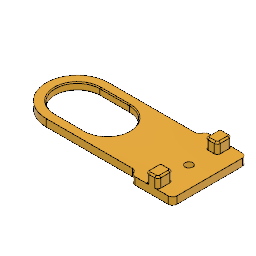
filament guide v6 (Autodesk Fusion 360 design; units mm, degrees)
Autodesk Fusion 360 part; units mm, degrees
sketch "Sketch1" plane through (0, 0, 0) normal (0, 1, 0) x (1, 0, 0)
  line L0 (0, 0) -> (-75, 0) construction
  circle A0 centre (-75, 0) radius 15
  circle A1 centre (-75, 0) radius 21
  circle A2 centre (-55, 0) radius 15
  line L1 (14, -25) -> (-14, -25)
  line L2 (-14, -25) -> (-14, 25)
  line L3 (-14, 25) -> (14, 25)
  line L4 (14, 25) -> (14, -25)
  line L5 (14, -25) -> (-14, 25) construction
  line L6 (-14, -25) -> (14, 25) construction
  line L7 (-14, 21) -> (-75, 21)
  line L8 (-14, -21) -> (-75, -21)
  line L9 (-75, 15) -> (-55, 15)
  line L10 (-75, -15) -> (-55, -15)
  circle A3 centre (0, 0) radius 2.6
  line L11 (15, -29.9919) -> (-15, -29.9919) construction
  line L12 (-15, -29.9919) -> (-15, 29.9919) construction
  line L13 (-15, 29.9919) -> (15, 29.9919) construction
  line L14 (15, 29.9919) -> (15, -29.9919) construction
  line L15 (15, -29.9919) -> (-15, 29.9919) construction
  line L16 (-15, -29.9919) -> (15, 29.9919) construction
  line L17 (-4.05, -25) -> (4.05, -25)
  line L18 (4.05, -25) -> (4.05, -15)
  line L19 (4.05, -15) -> (-4.05, -15)
  line L20 (-4.05, -15) -> (-4.05, -25)
  line L21 (0, -25) -> (0, 25) construction
  line L22 (4.05, 25) -> (4.05, 15)
  line L23 (4.05, 15) -> (-4.05, 15)
  line L24 (-4.05, 25) -> (4.05, 25)
  line L25 (-4.05, 15) -> (-4.05, 25)
  point P0 (-90, 0)
  point P1 (-40, 0)
  dimension "d1" = 30
  dimension "d3" = 30
  dimension "d4" = 42
  dimension "d5" = 50
  dimension "d6" = 28
  dimension "d9" = 5.2
  dimension "d20" = 30
  dimension "d23" = 75
  dimension "d24" = 25
  dimension "d25" = 10
  dimension "d26" = 8.1
  constraint horizontal L0
  constraint coincident A3.centre L0
  constraint coincident L0 A0.centre
  constraint coincident L0 A2.centre
  constraint perpendicular L1 L2
  constraint parallel L1 L3
  constraint parallel L2 L4
  constraint horizontal L1
  constraint coincident L5 L0.start
  constraint coincident L6 L0.start
  constraint coincident L0.start A3.centre
  constraint coincident L2 L7.start
  constraint coincident A1 L7.end
  constraint tangent A1 L7
  constraint horizontal L7
  constraint coincident L2 L8.start
  constraint coincident A1 L8.end
  constraint tangent A1 L8
  constraint horizontal L8
  constraint coincident A0 L9.start
  constraint coincident A2 L9.end
  constraint tangent A2 L9
  constraint horizontal L9
  constraint coincident A0 L10.start
  constraint coincident A2 L10.end
  constraint tangent A2 L10
  constraint horizontal L10
  constraint coincident A0 P0
  constraint coincident A2 P1
  constraint coincident L0 P0
  constraint coincident L0 P1
  constraint coincident L0.end A0.centre
  constraint perpendicular L11 L12
  constraint parallel L11 L13
  constraint parallel L12 L14
  constraint horizontal L11
  constraint coincident L15 L0.start
  constraint coincident L16 L0.start
  constraint concentric A0 A1
  constraint horizontal L17
  constraint vertical L18
  constraint horizontal L19
  constraint vertical L20
  constraint midpoint L1 L21.start
  constraint midpoint L3 L21.end
  constraint midpoint L17 L21.start
  constraint symmetric L0 L17.start L24.start
  constraint symmetric L0 L17.end L22.start
  constraint symmetric L0 L18.end L22.end
  constraint symmetric L0 L19.end L23.end
  measures "d1" diameter of A2
  measures "d3" diameter of A0
  measures "d4" diameter of A1
  measures "d5" distance of L1.end L2.end
  measures "d6" distance of L2.end L3.end
  measures "d9" diameter of A3
  measures "d20" distance of L11.start L11.end
  measures "d23" distance of P0 L12
  measures "d24" distance of P1 L12
  measures "d25" distance of L17.end L18.end
  measures "d26" distance of L17.start L17.end
extrude "Extrude1" add sketch "Sketch1" along normal blind 5 contours A0 A1 L9 L10 | A1 A2 L2 L7 L8 L9 L10 | L1 L2 L3 L4 L18 L19 L20 L22 L23 L25 | L3 L22 L23 L24 L25 | L1 L17 L18 L19 L20
extrude "Extrude2" add sketch "Sketch1" along normal blind 7 from surface at 5 contours L3 L22 L23 L24 L25 | L1 L17 L18 L19 L20
fillet "Fillet1" radius 3 6 edges at (14, 2.5, -25) (-14, 2.5, -25) (-14, 2.5, 25) (14, 2.5, 25) (-14, 2.5, -21) (-14, 2.5, 21)
chamfer "Chamfer1" distance 0.6 angle 45 8 edges at (-65, 5, -15) (-40, 5, 0) (-65, 5, 15) (-90, 5, 0) (-90, 0, 0) (-65, 0, -15) (-40, 0, 0) (-65, 0, 15)
fillet "Fillet2" radius 2 8 edges at (4.05, 8.5, 15) (-4.05, 8.5, 15) (-4.05, 8.5, 25) (4.05, 8.5, 25) (4.05, 8.5, -25) (4.05, 8.5, -15) (-4.05, 8.5, -15) (-4.05, 8.5, -25)
chamfer "Chamfer2" distance 1 angle 45 16 edges at (3.4642, 12, -24.4142) (0, 12, -25) (-3.4642, 12, -24.4142) (-4.05, 12, -20) (-3.4642, 12, -15.5858) (0, 12, -15) (3.4642, 12, -15.5858) (4.05, 12, -20) (-3.4642, 12, 15.5858) (-4.05, 12, 20) (-3.4642, 12, 24.4142) (0, 12, 25) (3.4642, 12, 24.4142) (4.05, 12, 20) (3.4642, 12, 15.5858) (0, 12, 15)
equation "d2 = d1 + ( 2 * 4 ) * 1 mm"
equation "d3 = d1"
equation "d4 = d1 + ( 2 * 6 ) * 1 mm"
